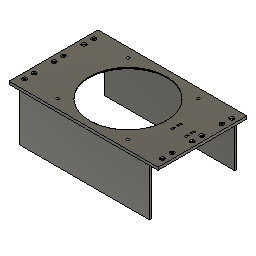
shared_fan_plate (Autodesk Fusion 360 design; units mm, degrees)
part number: 2026-08-27-12-22-23-518
Autodesk Fusion 360 part; units mm, degrees
sketch "Sketch: plate" plane through (0, 0, 0) normal (0, 0, 1) x (1, 0, 0)
  line L0 (-111, 0.4) -> (111, 0.4)
  line L1 (111, 0.4) -> (111, 132.95)
  line L2 (111, 132.95) -> (-111, 132.95)
  line L3 (-111, 132.95) -> (-111, 0.4)
extrude "Plate" add sketch "Sketch: plate" along normal blind 4
sketch "Sketch: duct walls" plane through (0, 0, 0) normal (0, 0, 1) x (1, 0, 0)
  line L0 (-96.72, 2.1) -> (96.72, 2.1)
  line L1 (96.72, 2.1) -> (96.72, 4.3)
  line L2 (96.72, 4.3) -> (-96.72, 4.3)
  line L3 (-96.72, 4.3) -> (-96.72, 2.1)
  line L4 (-96.72, 129.05) -> (96.72, 129.05)
  line L5 (96.72, 129.05) -> (96.72, 131.25)
  line L6 (96.72, 131.25) -> (-96.72, 131.25)
  line L7 (-96.72, 131.25) -> (-96.72, 129.05)
extrude "Duct walls" add sketch "Sketch: duct walls" against normal blind 72
sketch "Sketch: openings and holes" plane through (0, 0, 0) normal (0, 0, 1) x (1, 0, 0)
  circle A0 centre (0, 66.675) radius 57
  circle A1 centre (-52.5, 14.175) radius 2.25
  circle A2 centre (-52.5, 119.175) radius 2.25
  circle A3 centre (52.5, 14.175) radius 2.25
  circle A4 centre (52.5, 119.175) radius 2.25
  circle A5 centre (-102.82, 15) radius 1.7
  circle A6 centre (-102.82, 29.45) radius 1.7
  circle A7 centre (-102.82, 59.45) radius 1.7
  circle A8 centre (-102.82, 73.9) radius 1.7
  circle A9 centre (-102.82, 103.9) radius 1.7
  circle A10 centre (-102.82, 118.35) radius 1.7
  circle A11 centre (102.82, 15) radius 1.7
  circle A12 centre (102.82, 29.45) radius 1.7
  circle A13 centre (102.82, 59.45) radius 1.7
  circle A14 centre (102.82, 73.9) radius 1.7
  circle A15 centre (102.82, 103.9) radius 1.7
  circle A16 centre (102.82, 118.35) radius 1.7
extrude "Openings and holes" cut sketch "Sketch: openings and holes" along normal blind 4
sketch "Sketch: tie slots" plane through (0, 0, 0) normal (0, 0, 1) x (1, 0, 0)
  line L0 (70.75, 59.425) -> (73.25, 59.425)
  line L1 (73.25, 59.425) -> (73.25, 64.425)
  line L2 (73.25, 64.425) -> (70.75, 64.425)
  line L3 (70.75, 64.425) -> (70.75, 59.425)
  line L4 (70.75, 68.925) -> (73.25, 68.925)
  line L5 (73.25, 68.925) -> (73.25, 73.925)
  line L6 (73.25, 73.925) -> (70.75, 73.925)
  line L7 (70.75, 73.925) -> (70.75, 68.925)
  line L8 (90.75, 59.425) -> (93.25, 59.425)
  line L9 (93.25, 59.425) -> (93.25, 64.425)
  line L10 (93.25, 64.425) -> (90.75, 64.425)
  line L11 (90.75, 64.425) -> (90.75, 59.425)
  line L12 (90.75, 68.925) -> (93.25, 68.925)
  line L13 (93.25, 68.925) -> (93.25, 73.925)
  line L14 (93.25, 73.925) -> (90.75, 73.925)
  line L15 (90.75, 73.925) -> (90.75, 68.925)
extrude "Tie slots" cut sketch "Sketch: tie slots" along normal blind 4
ref_plane "WorkPlane1" through (0, 0, 4) normal (0, 0, 1) x (1, 0, 0)
sketch "Sketch: head counterbores" plane through (0, 0, 4) normal (0, 0, 1) x (1, 0, 0)
  circle A0 centre (-102.82, 15) radius 3.25
  circle A1 centre (-102.82, 29.45) radius 3.25
  circle A2 centre (-102.82, 59.45) radius 3.25
  circle A3 centre (-102.82, 73.9) radius 3.25
  circle A4 centre (-102.82, 103.9) radius 3.25
  circle A5 centre (-102.82, 118.35) radius 3.25
  circle A6 centre (102.82, 15) radius 3.25
  circle A7 centre (102.82, 29.45) radius 3.25
  circle A8 centre (102.82, 59.45) radius 3.25
  circle A9 centre (102.82, 73.9) radius 3.25
  circle A10 centre (102.82, 103.9) radius 3.25
  circle A11 centre (102.82, 118.35) radius 3.25
extrude "Head counterbores" cut sketch "Sketch: head counterbores" against normal blind 2
chamfer "Inlet chamfer" distance 3 angle 45 1 edges at (-53.1427, 46.0629, 0)
named bodies: "Shared Duct Fan Plate"
